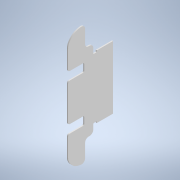
# Autodesk Inventor part: motherCATboard
Saved by Autodesk Inventor 2022 (Build 260153000, 153)
## iProperties
Created: 2024-07-28
Part Number: motherCATboard
Material: Типовые
Document SubType Name: Modeling
Designer: Капустяник Андрей
Density: 1 g/cm^3
Appearance: По умолчанию
Author: Капустяник Андрей
Autodesk Inventor part; units mm, degrees
ref_plane "YZ Plane" through (0, 0, 0) normal (1, 0, 0) x (0, 1, 0)
ref_plane "XZ Plane" through (0, 0, 0) normal (0, 1, 0) x (-1, 0, 0)
ref_plane "XY Plane" through (0, 0, 0) normal (0, 0, 1) x (1, 0, 0)
sketch "Эскиз1" plane through (0, 0, 0) normal (1, 0, 0) x (0, 1, 0)
  line L0 (40, 25) -> (-40, 25)
  line L1 (-40, 25) -> (-40, -25)
  line L2 (-40, -25) -> (40, -25)
  line L3 (40, -25) -> (40, 25)
  line L4 (40, 25) -> (-40, -25) construction
  line L5 (-40, 25) -> (40, -25) construction
  line L6 (40.5, -32.055) -> (-40.5, -32.055) projected
  line L7 (-17.0687, -48) -> (-17.0687, -49) projected
  line L8 (-17.0687, -49) -> (-19.4514, -49) projected
  line L9 (-19.4514, -49) -> (-19.4514, -59) projected
  line L10 (-19.4514, -59) -> (-17.0687, -59) projected
  line L11 (-17.0687, -59) -> (-17.0687, -74) projected
  line L12 (-17.0687, -74) -> (-39.5, -74) projected
  line L13 (-43.5, -31.055) -> (-43.5, 25) projected
  line L14 (-43.5, 25) -> (43.5, 25) projected
  line L15 (43.5, 25) -> (43.5, -31.055) projected
  line L16 (39.5, -74) -> (5.9221, -74) projected
  line L17 (5.9221, -74) -> (5.9221, -48) projected
  line L18 (5.9221, -48) -> (-17.0687, -48) projected
  line L19 (-43.5, -32.055) -> (43.5, -32.055)
  line L20 (43.5, -32.055) -> (43.5, 25)
  line L21 (43.5, 25) -> (-43.5, 25)
  line L22 (-43.5, 25) -> (-43.5, -32.055)
  line L23 (39.5, -30.555) -> (-39.5, -30.555) projected
  line L24 (-43.5, -30.255) -> (43.5, -30.255)
  line L25 (-39.5, -74) -> (-39.5, -31.055) projected
  line L26 (-39.5, -31.055) -> (-43.5, -31.055) projected
  line L27 (43.5, -31.055) -> (39.5, -31.055) projected
  line L28 (39.5, -31.055) -> (39.5, -74) projected
  point P0 (0, 0)
  point P1 (-43.5, -30.255)
  point P2 (43.5, -30.255)
  dimension "d0" = 80
  dimension "d1" = 50
  dimension "d4" = 0.3
  constraints: 22 end point, 5 parallel, 3 point on line, 2 horizontal, 2 midpoint, 2 perpendicular, 1 collinear
  measures "d0" distance of L2.end L1.end
  measures "d1" distance of L1.end L0.end
  measures "d4" distance between parallel lines of L23 L24
extrude "Выдавливание1" add sketch "Эскиз1" along normal blind 1.2 contours L3 L2 L1 L0 | L14 L15 L24 L13 L1 L2 L3
sketch "Эскиз2" plane through (0, 0, 0) normal (-1, 0, 0) x (0, 0, 1)
  line L0 (7.3, -28.9) -> (7.3, -22.3) projected
  arc A0 (8.3, -21.3) -> (7.3, -22.3) centre (8.3, -22.3) ccw projected
  line L1 (8.3, -21.3) -> (19, -21.3) projected
  line L2 (19, 21.3) -> (8.3, 21.3) projected
  arc A1 (7.3, 22.3) -> (8.3, 21.3) centre (8.3, 22.3) ccw projected
  line L3 (7.3, 22.3) -> (7.3, 28.9) projected
  line L4 (7, -43.5) -> (7, -22.3)
  arc A2 (8.3, -21) -> (7, -22.3) centre (8.3, -22.3) ccw
  line L5 (8.3, -21) -> (25, -21)
  line L6 (25, 21) -> (8.3, 21)
  arc A3 (7, 22.3) -> (8.3, 21) centre (8.3, 22.3) ccw
  line L7 (7, 22.3) -> (7, 43.5)
  line L8 (25, 43.5) -> (25, -43.5) projected
  line L9 (-30.255, 43.5) -> (25, 43.5) projected
  line L10 (25, -43.5) -> (-30.255, -43.5) projected
  line L11 (-30.255, -43.5) -> (-30.255, 43.5) projected
  line L12 (19, -29.9) -> (8.3, -29.9) projected
  arc A4 (7.3, -28.9) -> (8.3, -29.9) centre (8.3, -28.9) ccw projected
  line L13 (8.3, 29.9) -> (19, 29.9) projected
  arc A5 (8.3, 29.9) -> (7.3, 28.9) centre (8.3, 28.9) ccw projected
  line L14 (19, 21) -> (8.3, 21)
  arc A6 (7, 22.3) -> (8.3, 21) centre (8.3, 22.3) ccw
  line L15 (7, 22.3) -> (7, 28.9)
  arc A7 (8.3, 30.2) -> (7, 28.9) centre (8.3, 28.9) ccw
  line L16 (8.3, 30.2) -> (25, 30.2)
  line L17 (25, -30.2) -> (8.3, -30.2)
  arc A8 (7, -28.9) -> (8.3, -30.2) centre (8.3, -28.9) ccw
  line L18 (7, -28.9) -> (7, -22.3)
  arc A9 (8.3, -21) -> (7, -22.3) centre (8.3, -22.3) ccw
  line L19 (8.3, -21) -> (19, -21)
  point P0 (7, -28.9)
  dimension "d15" = 0.3
  dimension "d16" = 0.3
  dimension "d26" = 0.3
  dimension "d27" = 0.3
  constraints: 20 end point, 12 point on circle, 6 centre point, 6 point on line, 12 other
  measures "d15" distance between parallel lines of L0 L4
  measures "d16" radial gap between concentric circles of A1 A3
  measures "d26" radial gap between concentric circles of A5 A7
  measures "d27" distance between parallel lines of L12 L17
extrude "Выдавливание2" cut sketch "Эскиз2" against normal blind 10 contours L4 A2 L5 L8 L17 A8 | L6 A3 L7 A7 L16 L8
sketch "Эскиз4" plane through (0, 0, 0) normal (-1, 0, 0) x (0, 0, 1)
  line L0 (-4.0814, -35.48) -> (-4.0814, -33.727) projected
  line L1 (-4.0814, 33.727) -> (-4.0814, 35.48) projected
  line L2 (25, -43.5) -> (-30.255, -43.5) projected
  line L3 (7, -28.9) -> (7, -22.3) projected
  line L4 (25, 21) -> (8.3, 21) projected
  arc A0 (7, 22.3) -> (8.3, 21) centre (8.3, 22.3) ccw projected
  line L5 (7, 22.3) -> (7, 28.9) projected
  line L6 (-30.255, 43.5) -> (25, 43.5) projected
  line L7 (-30.255, -43.5) -> (-30.255, 43.5) projected
  line L8 (25, -43.5) -> (-30.255, -43.5) projected
  line L9 (7, -28.9) -> (7, -22.3) projected
  arc A1 (8.3, -21) -> (7, -22.3) centre (8.3, -22.3) ccw projected
  line L10 (8.3, -21) -> (25, -21) projected
  line L11 (25, 21) -> (25, -21) projected
  line L12 (-25.0814, -35) -> (4.9186, -35)
  line L13 (4.9186, -35) -> (4.9186, 35)
  line L14 (4.9186, 35) -> (-25.0814, 35)
  line L15 (-25.0814, 35) -> (-25.0814, -35)
  line L16 (-30.255, -43.5) -> (-30.255, 43.5) projected
  line L17 (-30.255, 0) -> (25, 0)
  line L18 (4.9186, -35) -> (-3.0814, -35)
  line L19 (-3.0814, -35) -> (-3.0814, -33.3)
  line L20 (-3.0814, -33.3) -> (-7.0814, -33.3)
  line L21 (-7.0814, -33.3) -> (-7.0814, -35)
  line L22 (-3.0814, 35) -> (-3.0814, 33.3)
  line L23 (-3.0814, 33.3) -> (-7.0814, 33.3)
  line L24 (-7.0814, 33.3) -> (-7.0814, 35)
  line L25 (-3.0814, -35) -> (-3.0814, -43.5)
  line L26 (-3.0814, 35) -> (-3.0814, 43.5)
  line L27 (-30.255, 43.5) -> (7, 43.5) projected
  line L28 (25, -30.2) -> (8.3, -30.2) projected
  arc A2 (7, -28.9) -> (8.3, -30.2) centre (8.3, -28.9) ccw projected
  arc A3 (8.3, 30.2) -> (7, 28.9) centre (8.3, 28.9) ccw projected
  line L29 (8.3, 30.2) -> (25, 30.2) projected
  line L30 (25, 43.5) -> (25, 30.2) projected
  line L31 (25, -30.2) -> (25, -43.5) projected
  point P0 (0, 0)
  point P1 (7, -43.5)
  point P2 (-25.0814, 0)
  point P3 (-7.0814, 35)
  point P4 (-3.0814, 43.5)
  point P5 (-3.0814, -43.5)
  dimension "d17" = 70
  dimension "d18" = 30
  dimension "d19" = 9
  dimension "d20" = 8
  dimension "d21" = 1.7
  dimension "d22" = 4
  constraints: 28 end point, 6 point on line, 5 perpendicular, 4 symmetric about line, 3 midpoint, 2 parallel, 1 horizontal
  measures "d17" distance of L13.end L12.end
  measures "d18" distance between parallel lines of L13 L15
  measures "d19" distance between parallel lines of L13 L0
  measures "d20" distance of L12.end L18.end
  measures "d21" distance of L18.end L19.end
  measures "d22" distance of L19.end L20.end
extrude "Выдавливание4" cut sketch "Эскиз4" against normal blind 10 contours L2 L7 L17 L15 L12 L25 | L12 L21 L20 L19 | L7 L6 L26 L14 L15 L17 | L22 L23 L24 L14
fillet "Сопряжение3" radius 0.8 4 edges at (0.6, -33.3, -7.0814) (0.6, -33.3, -3.0814) (0.6, 33.3, -7.0814) (0.6, 33.3, -3.0814)
sketch "Эскиз5" plane through (0, 0, 0) normal (-1, 0, 0) x (0, 0, 1)
  line L0 (-3.0814, -34.1) -> (-3.0814, -43.5)
  line L1 (25, -43.5) -> (-3.0814, -43.5)
  line L2 (25, -30.2) -> (25, -43.5)
  line L3 (25, -30.2) -> (8.3, -30.2)
  arc A0 (7, -28.9) -> (8.3, -30.2) centre (8.3, -28.9) ccw
  line L4 (7, -28.9) -> (7, -22.3)
  arc A1 (8.3, -21) -> (7, -22.3) centre (8.3, -22.3) ccw
  line L5 (8.3, -21) -> (25, -21)
  line L6 (25, 21) -> (25, -21)
  line L7 (25, 21) -> (8.3, 21)
  arc A2 (7, 22.3) -> (8.3, 21) centre (8.3, 22.3) ccw
  line L8 (7, 22.3) -> (7, 28.9)
  arc A3 (8.3, 30.2) -> (7, 28.9) centre (8.3, 28.9) ccw
  line L9 (8.3, 30.2) -> (25, 30.2)
  line L10 (25, 43.5) -> (25, 30.2)
  line L11 (-3.0814, 43.5) -> (25, 43.5)
  line L12 (-3.0814, 43.5) -> (-3.0814, 34.1)
  arc A4 (-3.8814, 33.3) -> (-3.0814, 34.1) centre (-3.8814, 34.1) ccw
  line L13 (-3.8814, 33.3) -> (-6.2814, 33.3)
  arc A5 (-7.0814, 34.1) -> (-6.2814, 33.3) centre (-6.2814, 34.1) ccw
  line L14 (-7.0814, 34.1) -> (-7.0814, 35)
  line L15 (-7.0814, 35) -> (-25.0814, 35)
  line L16 (-25.0814, 35) -> (-25.0814, -35)
  line L17 (-25.0814, -35) -> (-7.0814, -35)
  line L18 (-7.0814, -35) -> (-7.0814, -34.1)
  arc A6 (-6.2814, -33.3) -> (-7.0814, -34.1) centre (-6.2814, -34.1) ccw
  line L19 (-6.2814, -33.3) -> (-3.8814, -33.3)
  arc A7 (-3.0814, -34.1) -> (-3.8814, -33.3) centre (-3.8814, -34.1) ccw
  line L20 (-104.4698, -3.8) -> (-104.4698, 15.7)
  arc A8 (-101.4698, 18.7) -> (-104.4698, 15.7) centre (-101.4698, 15.7) ccw
  line L21 (-101.4698, 18.7) -> (-87.7061, 18.7)
  arc A9 (-84.7061, 15.7) -> (-87.7061, 18.7) centre (-87.7061, 15.7) ccw
  line L22 (-84.7061, 15.7) -> (-84.7061, -3.8)
  arc A10 (-87.7061, -6.8) -> (-84.7061, -3.8) centre (-87.7061, -3.8) ccw
  line L23 (-87.7061, -6.8) -> (-101.4698, -6.8)
  arc A11 (-104.4698, -3.8) -> (-101.4698, -6.8) centre (-101.4698, -3.8) ccw
  line L24 (6.7, -28.4) -> (6.7, -21.6)
  line L25 (6.7, -21.6) -> (20.6, -21.6)
  line L26 (20.6, -21.6) -> (20.6, -28.4)
  line L27 (20.6, -28.4) -> (6.7, -28.4)
  line L28 (6.7, 28.4) -> (20.6, 28.4)
  line L29 (20.6, 28.4) -> (20.6, 21.6)
  line L30 (20.6, 21.6) -> (6.7, 21.6)
  line L31 (6.7, 21.6) -> (6.7, 28.4)
  circle A12 centre (-85.1704, -33.954) radius 1.5
  circle A13 centre (-105.6714, -23.0046) radius 1.5
  circle A14 centre (-105.6714, 23.0046) radius 1.5
  circle A15 centre (-85.1704, 33.954) radius 1.5
  line L32 (-17.8533, 40.5) -> (2.75, 40.5)
  line L33 (2.75, 40.5) -> (2.75, 25.5)
  line L34 (2.75, 25.5) -> (-17.8533, 25.5)
  line L35 (-17.8533, 25.5) -> (-17.8533, 40.5)
  line L36 (-77.0704, 40) -> (-77.0704, 43.5)
  line L37 (-77.0704, 43.5) -> (-114, 43.5)
  line L38 (-114, 43.5) -> (-114, 62.7947)
  line L39 (-114, 62.7947) -> (6, 62.7947)
  line L40 (6, 62.7947) -> (6, 43.5)
  line L41 (6, 43.5) -> (-32.055, 43.5)
  line L42 (-32.055, 43.5) -> (-32.055, -43.5)
  line L43 (-32.055, -43.5) -> (6, -43.5)
  line L44 (6, -43.5) -> (6, -62.7947)
  line L45 (6, -62.7947) -> (-114, -62.7947)
  line L46 (-114, -62.7947) -> (-114, -43.5)
  line L47 (-114, -43.5) -> (-77.0704, -43.5)
  line L48 (-77.0704, -43.5) -> (-77.0704, -40)
  line L49 (-77.0704, -40) -> (-76.0704, -40)
  line L50 (-76.0704, -40) -> (-76.0704, -27.6138)
  line L51 (-76.0704, -27.6138) -> (-77.1963, -27.6138)
  line L52 (-77.1963, -27.6138) -> (-77.1963, -10.238)
  line L53 (-77.1963, -10.238) -> (-76.0704, -10.238)
  line L54 (-76.0704, -10.238) -> (-76.0704, -5)
  line L55 (-76.0704, -5) -> (-79.0704, -5)
  line L56 (-79.0704, -5) -> (-79.0704, 5)
  line L57 (-79.0704, 5) -> (-76.0704, 5)
  line L58 (-76.0704, 5) -> (-76.0704, 10.238)
  line L59 (-76.0704, 10.238) -> (-77.1963, 10.238)
  line L60 (-77.1963, 10.238) -> (-77.1963, 27.6138)
  line L61 (-77.1963, 27.6138) -> (-76.0704, 27.6138)
  line L62 (-76.0704, 27.6138) -> (-76.0704, 40)
  line L63 (-76.0704, 40) -> (-77.0704, 40)
  circle A16 centre (-83.5, -25.5) radius 1.25
  circle A17 centre (-24.5, 25.5) radius 1.25
  circle A18 centre (-24.5, -25.5) radius 1.25
  circle A19 centre (-83.5, 25.5) radius 1.25
  arc A20 (23, 6) -> (25, 8) centre (23, 8) ccw
  line L64 (25, 52.7636) -> (25, 8)
  spline S0 degree 4 poles (17.7798, 64.1091) (21.0942, 61.9787) (24.3169, 57.93) (25, 55.716) (25, 52.7636) knots 0 0 0 0 0 1 1 1 1 1
  spline S1 degree 2 poles (1, 66.7947) (12.9746, 67.1977) (17.7798, 64.1091) knots 0 0 0 0.595743 0.595743 0.595743
  line L65 (-109, 66.7947) -> (1, 66.7947)
  spline S2 degree 2 poles (-125.7798, 64.1091) (-120.9746, 67.1977) (-109, 66.7947) knots -0.595743 -0.595743 -0.595743 0 0 0
  spline S3 degree 4 poles (-125.7798, 64.1091) (-129.0942, 61.9787) (-132.3169, 57.93) (-133, 55.716) (-133, 52.7636) knots 0 0 0 0 0 1 1 1 1 1
  line L66 (-133, 52.7636) -> (-133, 5)
  line L67 (-133, 5) -> (-114, 5)
  line L68 (-114, 5) -> (-114, -5)
  line L69 (-114, -5) -> (-133, -5)
  line L70 (-133, -5) -> (-133, -52.7636)
  spline S4 degree 4 poles (-125.7798, -64.1091) (-129.0942, -61.9787) (-132.3169, -57.93) (-133, -55.716) (-133, -52.7636) knots 0 0 0 0 0 1 1 1 1 1
  spline S5 degree 2 poles (-109, -66.7947) (-120.9746, -67.1977) (-125.7798, -64.1091) knots 0 0 0 0.595743 0.595743 0.595743
  line L71 (1, -66.7947) -> (-109, -66.7947)
  spline S6 degree 2 poles (1, -66.7947) (12.9746, -67.1977) (17.7798, -64.1091) knots 0 0 0 0.595743 0.595743 0.595743
  spline S7 degree 4 poles (17.7798, -64.1091) (17.7903, -64.1023) (17.8008, -64.0955) (17.8113, -64.0887) (17.8219, -64.0819) knots 0 0 0 0 0 1 1 1 1 1
  spline S8 degree 4 poles (19.0101, -63.2209) (18.7505, -63.4512) (18.4659, -63.6716) (18.1563, -63.8819) (17.8219, -64.0819) knots 0 0 0 0 0 1 1 1 1 1
  spline S9 degree 4 poles (19.0101, -63.2209) (21.9352, -60.8863) (24.439, -57.5084) (25, -55.4392) (25, -52.7636) knots 0.093747 0.093747 0.093747 0.093747 0.093747 1 1 1 1 1
  line L72 (25, -8) -> (25, -52.7636)
  arc A21 (25, -8) -> (23, -6) centre (23, -8) ccw
  line L73 (23, -6) -> (9.1467, -6)
  arc A22 (8.1467, -5) -> (9.1467, -6) centre (9.1467, -5) ccw
  line L74 (8.1467, -5) -> (8.1467, 5)
  arc A23 (9.1467, 6) -> (8.1467, 5) centre (9.1467, 5) ccw
  line L75 (9.1467, 6) -> (23, 6)
  line L76 (6, -66.8003) -> (6, 66.8003)
  point P0 (0, 0)
  constraints: 2 end point, 1 collinear, 1 vertical, 2 other
extrude "Выдавливание5" add sketch "Эскиз5" against normal blind 1.2 contours L1 L72 S9 S8 S7 S6 L76 L44 | L40 L76 S1 S0 L64 L11
fillet "Сопряжение4" radius 4 6 edges at (0.6, 43.5, 6) (0.6, 43.5, -3.0814) (0.6, 66.8003, 6) (0.6, -43.5, 6) (0.6, -43.5, -3.0814) (0.6, -66.8003, 6)
fillet "Сопряжение5" radius 2 4 edges at (0.6, -30.2, 25) (0.6, -21, 25) (0.6, 21, 25) (0.6, 30.2, 25)
